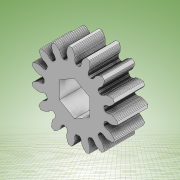
# Autodesk Inventor part: Piñon1
Saved by Autodesk Inventor 2022 (Build 260153000, 153)
## iProperties
Created: 2022-03-08
Part Number: Piñon1
Material: Genérico
Document SubType Name: Modeling
Designer: Marco
Density: 1 g/cm^3
Appearance: Valor por defecto
Author: Marco
Autodesk Inventor part; units mm, degrees
ref_plane "YZ Plane" through (0, 0, 0) normal (1, 0, 0) x (0, 1, 0)
ref_plane "XZ Plane" through (0, 0, 0) normal (0, 1, 0) x (-1, 0, 0)
ref_plane "XY Plane" through (0, 0, 0) normal (0, 0, 1) x (1, 0, 0)
sketch "Boceto1" plane through (0, 0, 0) normal (0, 0, 1) x (1, 0, 0)
  line L0 (7.7848, 3.0032) -> (7.6735, 2.8594)
  line L1 (7.6735, 2.8594) -> (7.565, 2.7306)
  line L2 (7.565, 2.7306) -> (7.4594, 2.6156)
  line L3 (7.4594, 2.6156) -> (7.3576, 2.5136)
  line L4 (7.3576, 2.5136) -> (7.2614, 2.4249)
  line L5 (7.2614, 2.4249) -> (7.1696, 2.3471)
  line L6 (7.1696, 2.3471) -> (7.0863, 2.2824)
  line L7 (7.0863, 2.2824) -> (7.01, 2.228)
  line L8 (7.01, 2.228) -> (6.8817, 2.1478)
  line L9 (6.8817, 2.1478) -> (6.7742, 2.0935)
  line L10 (6.7742, 2.0935) -> (6.6296, 2.0713)
  line L11 (6.6296, 2.0713) -> (6.4798, 2.0382)
  line L12 (6.4798, 2.0382) -> (6.3445, 1.9967)
  line L13 (6.3445, 1.9967) -> (6.2241, 1.948)
  line L14 (6.2241, 1.948) -> (6.119, 1.8933)
  line L15 (6.119, 1.8933) -> (6.0294, 1.8338)
  line L16 (6.0294, 1.8338) -> (5.9556, 1.7706)
  line L17 (5.9556, 1.7706) -> (5.9246, 1.738)
  line L18 (5.9246, 1.738) -> (5.8976, 1.705)
  line L19 (5.8976, 1.705) -> (5.8746, 1.6717)
  line L20 (5.8746, 1.6717) -> (5.8555, 1.6382)
  line L21 (5.8555, 1.6382) -> (5.8404, 1.6048)
  line L22 (5.8404, 1.6048) -> (5.8293, 1.5715)
  line L23 (5.8293, 1.5715) -> (5.8221, 1.5384)
  line L24 (5.8221, 1.5384) -> (5.8189, 1.5059)
  line L25 (5.8189, 1.5059) -> (5.8195, 1.474)
  line L26 (5.8195, 1.474) -> (5.8258, 1.4351)
  line L27 (5.8258, 1.4351) -> (5.8688, 1.2477)
  line L28 (5.8688, 1.2477) -> (5.9058, 1.0589)
  line L29 (5.9058, 1.0589) -> (5.9159, 1.0209)
  line L30 (5.9159, 1.0209) -> (5.9283, 0.9915)
  line L31 (5.9283, 0.9915) -> (5.9445, 0.9631)
  line L32 (5.9445, 0.9631) -> (5.9644, 0.9358)
  line L33 (5.9644, 0.9358) -> (5.9882, 0.9099)
  line L34 (5.9882, 0.9099) -> (6.0156, 0.8855)
  line L35 (6.0156, 0.8855) -> (6.0466, 0.8627)
  line L36 (6.0466, 0.8627) -> (6.0812, 0.8416)
  line L37 (6.0812, 0.8416) -> (6.1193, 0.8224)
  line L38 (6.1193, 0.8224) -> (6.1608, 0.8053)
  line L39 (6.1608, 0.8053) -> (6.254, 0.7776)
  line L40 (6.254, 0.7776) -> (6.36, 0.7597)
  line L41 (6.36, 0.7597) -> (6.4783, 0.7524)
  line L42 (6.4783, 0.7524) -> (6.6081, 0.7569)
  line L43 (6.6081, 0.7569) -> (6.7485, 0.7741)
  line L44 (6.7485, 0.7741) -> (6.8988, 0.8048)
  line L45 (6.8988, 0.8048) -> (7.04, 0.8433)
  line L46 (7.04, 0.8433) -> (7.1603, 0.8374)
  line L47 (7.1603, 0.8374) -> (7.3101, 0.8164)
  line L48 (7.3101, 0.8164) -> (7.4019, 0.7977)
  line L49 (7.4019, 0.7977) -> (7.5044, 0.7724)
  line L50 (7.5044, 0.7724) -> (7.6198, 0.7388)
  line L51 (7.6198, 0.7388) -> (7.7438, 0.6969)
  line L52 (7.7438, 0.6969) -> (7.8783, 0.6451)
  line L53 (7.8783, 0.6451) -> (8.0216, 0.5829)
  line L54 (8.0216, 0.5829) -> (8.1731, 0.5095)
  line L55 (8.1731, 0.5095) -> (8.3334, 0.4231)
  line L56 (8.3334, 0.4231) -> (8.4936, 0.328)
  arc A0 (8.4936, -0.328) -> (8.4936, 0.328) centre (0, 0) ccw
  line L57 (8.4936, -0.328) -> (8.3332, -0.4231)
  line L58 (8.3332, -0.4231) -> (8.1741, -0.5093)
  line L59 (8.1741, -0.5093) -> (8.0225, -0.5827)
  line L60 (8.0225, -0.5827) -> (7.8793, -0.6449)
  line L61 (7.8793, -0.6449) -> (7.7448, -0.6966)
  line L62 (7.7448, -0.6966) -> (7.6208, -0.7384)
  line L63 (7.6208, -0.7384) -> (7.5053, -0.7721)
  line L64 (7.5053, -0.7721) -> (7.4028, -0.7973)
  line L65 (7.4028, -0.7973) -> (7.311, -0.8159)
  line L66 (7.311, -0.8159) -> (7.1612, -0.8369)
  line L67 (7.1612, -0.8369) -> (7.0409, -0.8427)
  line L68 (7.0409, -0.8427) -> (6.8997, -0.8042)
  line L69 (6.8997, -0.8042) -> (6.7494, -0.7734)
  line L70 (6.7494, -0.7734) -> (6.609, -0.7562)
  line L71 (6.609, -0.7562) -> (6.4792, -0.7517)
  line L72 (6.4792, -0.7517) -> (6.361, -0.7589)
  line L73 (6.361, -0.7589) -> (6.2549, -0.7768)
  line L74 (6.2549, -0.7768) -> (6.1617, -0.8044)
  line L75 (6.1617, -0.8044) -> (6.1202, -0.8216)
  line L76 (6.1202, -0.8216) -> (6.0821, -0.8407)
  line L77 (6.0821, -0.8407) -> (6.0475, -0.8618)
  line L78 (6.0475, -0.8618) -> (6.0164, -0.8846)
  line L79 (6.0164, -0.8846) -> (5.989, -0.909)
  line L80 (5.989, -0.909) -> (5.9653, -0.9349)
  line L81 (5.9653, -0.9349) -> (5.9453, -0.9621)
  line L82 (5.9453, -0.9621) -> (5.9291, -0.9906)
  line L83 (5.9291, -0.9906) -> (5.9167, -1.02)
  line L84 (5.9167, -1.02) -> (5.9066, -1.058)
  line L85 (5.9066, -1.058) -> (5.8696, -1.2467)
  line L86 (5.8696, -1.2467) -> (5.8265, -1.4342)
  line L87 (5.8265, -1.4342) -> (5.8202, -1.473)
  line L88 (5.8202, -1.473) -> (5.8196, -1.5049)
  line L89 (5.8196, -1.5049) -> (5.8228, -1.5375)
  line L90 (5.8228, -1.5375) -> (5.83, -1.5705)
  line L91 (5.83, -1.5705) -> (5.8411, -1.6038)
  line L92 (5.8411, -1.6038) -> (5.8561, -1.6373)
  line L93 (5.8561, -1.6373) -> (5.8752, -1.6708)
  line L94 (5.8752, -1.6708) -> (5.8982, -1.7041)
  line L95 (5.8982, -1.7041) -> (5.9252, -1.7371)
  line L96 (5.9252, -1.7371) -> (5.9562, -1.7697)
  line L97 (5.9562, -1.7697) -> (6.03, -1.8329)
  line L98 (6.03, -1.8329) -> (6.1196, -1.8925)
  line L99 (6.1196, -1.8925) -> (6.2246, -1.9472)
  line L100 (6.2246, -1.9472) -> (6.345, -1.9959)
  line L101 (6.345, -1.9959) -> (6.4803, -2.0374)
  line L102 (6.4803, -2.0374) -> (6.63, -2.0706)
  line L103 (6.63, -2.0706) -> (6.7746, -2.0929)
  line L104 (6.7746, -2.0929) -> (6.8822, -2.1472)
  line L105 (6.8822, -2.1472) -> (7.0104, -2.2275)
  line L106 (7.0104, -2.2275) -> (7.0867, -2.2818)
  line L107 (7.0867, -2.2818) -> (7.17, -2.3467)
  line L108 (7.17, -2.3467) -> (7.2617, -2.4244)
  line L109 (7.2617, -2.4244) -> (7.3579, -2.5131)
  line L110 (7.3579, -2.5131) -> (7.4597, -2.6152)
  line L111 (7.4597, -2.6152) -> (7.5652, -2.7303)
  line L112 (7.5652, -2.7303) -> (7.6737, -2.859)
  line L113 (7.6737, -2.859) -> (7.785, -3.0029)
  line L114 (7.785, -3.0029) -> (7.8927, -3.155)
  arc A1 (7.6259, -3.7544) -> (7.8927, -3.155) centre (0, 0) ccw
  line L115 (7.6259, -3.7544) -> (7.4407, -3.776)
  line L116 (7.4407, -3.776) -> (7.2594, -3.7895)
  line L117 (7.2594, -3.7895) -> (7.0911, -3.795)
  line L118 (7.0911, -3.795) -> (6.935, -3.7935)
  line L119 (6.935, -3.7935) -> (6.791, -3.7861)
  line L120 (6.791, -3.7861) -> (6.6607, -3.774)
  line L121 (6.6607, -3.774) -> (6.5416, -3.7578)
  line L122 (6.5416, -3.7578) -> (6.4376, -3.7392)
  line L123 (6.4376, -3.7392) -> (6.3462, -3.7189)
  line L124 (6.3462, -3.7189) -> (6.2008, -3.6772)
  line L125 (6.2008, -3.6772) -> (6.0885, -3.6336)
  line L126 (6.0885, -3.6336) -> (5.9752, -3.541)
  line L127 (5.9752, -3.541) -> (5.8504, -3.4518)
  line L128 (5.8504, -3.4518) -> (5.729, -3.379)
  line L129 (5.729, -3.379) -> (5.6123, -3.3222)
  line L130 (5.6123, -3.3222) -> (5.5013, -3.2807)
  line L131 (5.5013, -3.2807) -> (5.3972, -3.2539)
  line L132 (5.3972, -3.2539) -> (5.3008, -3.2413)
  line L133 (5.3008, -3.2413) -> (5.2559, -3.2401)
  line L134 (5.2559, -3.2401) -> (5.2133, -3.2421)
  line L135 (5.2133, -3.2421) -> (5.1731, -3.2473)
  line L136 (5.1731, -3.2473) -> (5.1355, -3.2555)
  line L137 (5.1355, -3.2555) -> (5.1005, -3.2667)
  line L138 (5.1005, -3.2667) -> (5.0683, -3.2807)
  line L139 (5.0683, -3.2807) -> (5.039, -3.2975)
  line L140 (5.039, -3.2975) -> (5.0126, -3.3168)
  line L141 (5.0126, -3.3168) -> (4.9893, -3.3387)
  line L142 (4.9893, -3.3387) -> (4.9646, -3.3693)
  line L143 (4.9646, -3.3693) -> (4.8541, -3.5267)
  line L144 (4.8541, -3.5267) -> (4.7386, -3.6805)
  line L145 (4.7386, -3.6805) -> (4.7171, -3.7134)
  line L146 (4.7171, -3.7134) -> (4.7035, -3.7423)
  line L147 (4.7035, -3.7423) -> (4.6932, -3.7734)
  line L148 (4.6932, -3.7734) -> (4.6863, -3.8064)
  line L149 (4.6863, -3.8064) -> (4.683, -3.8414)
  line L150 (4.683, -3.8414) -> (4.6831, -3.8781)
  line L151 (4.6831, -3.8781) -> (4.6869, -3.9164)
  line L152 (4.6869, -3.9164) -> (4.6944, -3.9562)
  line L153 (4.6944, -3.9562) -> (4.7057, -3.9974)
  line L154 (4.7057, -3.9974) -> (4.7207, -4.0397)
  line L155 (4.7207, -4.0397) -> (4.7625, -4.1275)
  line L156 (4.7625, -4.1275) -> (4.8201, -4.2183)
  line L157 (4.8201, -4.2183) -> (4.8939, -4.311)
  line L158 (4.8939, -4.311) -> (4.984, -4.4045)
  line L159 (4.984, -4.4045) -> (5.0908, -4.4974)
  line L160 (5.0908, -4.4974) -> (5.2141, -4.5885)
  line L161 (5.2141, -4.5885) -> (5.3372, -4.6677)
  line L162 (5.3372, -4.6677) -> (5.4134, -4.761)
  line L163 (5.4134, -4.761) -> (5.498, -4.8864)
  line L164 (5.498, -4.8864) -> (5.5455, -4.9671)
  line L165 (5.5455, -4.9671) -> (5.5953, -5.0602)
  line L166 (5.5953, -5.0602) -> (5.6475, -5.1685)
  line L167 (5.6475, -5.1685) -> (5.6994, -5.2887)
  line L168 (5.6994, -5.2887) -> (5.7509, -5.4233)
  line L169 (5.7509, -5.4233) -> (5.8005, -5.5713)
  line L170 (5.8005, -5.5713) -> (5.8473, -5.7331)
  line L171 (5.8473, -5.7331) -> (5.8905, -5.9097)
  line L172 (5.8905, -5.9097) -> (5.9271, -6.0925)
  arc A2 (5.4396, -6.5315) -> (5.9271, -6.0925) centre (0, 0) ccw
  line L173 (5.4396, -6.5315) -> (5.2616, -6.4759)
  line L174 (5.2616, -6.4759) -> (5.0905, -6.4145)
  line L175 (5.0905, -6.4145) -> (4.9345, -6.3511)
  line L176 (4.9345, -6.3511) -> (4.7924, -6.2862)
  line L177 (4.7924, -6.2862) -> (4.664, -6.221)
  line L178 (4.664, -6.221) -> (4.5499, -6.1568)
  line L179 (4.5499, -6.1568) -> (4.4476, -6.0936)
  line L180 (4.4476, -6.0936) -> (4.3602, -6.0343)
  line L181 (4.3602, -6.0343) -> (4.285, -5.9786)
  line L182 (4.285, -5.9786) -> (4.1691, -5.8814)
  line L183 (4.1691, -5.8814) -> (4.0842, -5.7958)
  line L184 (4.0842, -5.7958) -> (4.0184, -5.6652)
  line L185 (4.0184, -5.6652) -> (3.9406, -5.533)
  line L186 (3.9406, -5.533) -> (3.8594, -5.4171)
  line L187 (3.8594, -5.4171) -> (3.7759, -5.3177)
  line L188 (3.7759, -5.3177) -> (3.6914, -5.2346)
  line L189 (3.6914, -5.2346) -> (3.6071, -5.1678)
  line L190 (3.6071, -5.1678) -> (3.5242, -5.1171)
  line L191 (3.5242, -5.1171) -> (3.4836, -5.0977)
  line L192 (3.4836, -5.0977) -> (3.4439, -5.0822)
  line L193 (3.4439, -5.0822) -> (3.4051, -5.0706)
  line L194 (3.4051, -5.0706) -> (3.3673, -5.0628)
  line L195 (3.3673, -5.0628) -> (3.3309, -5.0588)
  line L196 (3.3309, -5.0588) -> (3.2957, -5.0585)
  line L197 (3.2957, -5.0585) -> (3.2621, -5.0619)
  line L198 (3.2621, -5.0619) -> (3.2302, -5.0689)
  line L199 (3.2302, -5.0689) -> (3.2, -5.0794)
  line L200 (3.2, -5.0794) -> (3.165, -5.0973)
  line L201 (3.165, -5.0973) -> (3, -5.1961)
  line L202 (3, -5.1961) -> (2.8319, -5.2896)
  line L203 (2.8319, -5.2896) -> (2.7989, -5.311)
  line L204 (2.7989, -5.311) -> (2.7747, -5.3318)
  line L205 (2.7747, -5.3318) -> (2.7527, -5.356)
  line L206 (2.7527, -5.356) -> (2.733, -5.3835)
  line L207 (2.733, -5.3835) -> (2.7157, -5.414)
  line L208 (2.7157, -5.414) -> (2.7009, -5.4476)
  line L209 (2.7009, -5.4476) -> (2.6888, -5.4842)
  line L210 (2.6888, -5.4842) -> (2.6794, -5.5236)
  line L211 (2.6794, -5.5236) -> (2.673, -5.5658)
  line L212 (2.673, -5.5658) -> (2.6695, -5.6106)
  line L213 (2.6695, -5.6106) -> (2.6719, -5.7077)
  line L214 (2.6719, -5.7077) -> (2.6876, -5.8141)
  line L215 (2.6876, -5.8141) -> (2.7173, -5.9288)
  line L216 (2.7173, -5.9288) -> (2.7617, -6.0509)
  line L217 (2.7617, -6.0509) -> (2.8214, -6.1791)
  line L218 (2.8214, -6.1791) -> (2.8971, -6.3126)
  line L219 (2.8971, -6.3126) -> (2.9773, -6.4349)
  line L220 (2.9773, -6.4349) -> (3.0089, -6.5512)
  line L221 (3.0089, -6.5512) -> (3.0352, -6.7002)
  line L222 (3.0352, -6.7002) -> (3.0458, -6.7932)
  line L223 (3.0458, -6.7932) -> (3.0534, -6.8985)
  line L224 (3.0534, -6.8985) -> (3.0571, -7.0187)
  line L225 (3.0571, -7.0187) -> (3.0555, -7.1496)
  line L226 (3.0555, -7.1496) -> (3.0478, -7.2935)
  line L227 (3.0478, -7.2935) -> (3.033, -7.449)
  line L228 (3.033, -7.449) -> (3.0099, -7.6157)
  line L229 (3.0099, -7.6157) -> (2.9775, -7.7947)
  line L230 (2.9775, -7.7947) -> (2.9366, -7.9766)
  arc A3 (2.3127, -8.1793) -> (2.9366, -7.9766) centre (0, 0) ccw
  line L231 (2.3127, -8.1793) -> (2.1727, -8.0562)
  line L232 (2.1727, -8.0562) -> (2.0413, -7.9305)
  line L233 (2.0413, -7.9305) -> (1.9247, -7.8092)
  line L234 (1.9247, -7.8092) -> (1.8213, -7.6921)
  line L235 (1.8213, -7.6921) -> (1.7305, -7.5802)
  line L236 (1.7305, -7.5802) -> (1.6523, -7.4752)
  line L237 (1.6523, -7.4752) -> (1.5846, -7.3758)
  line L238 (1.5846, -7.3758) -> (1.5289, -7.2862)
  line L239 (1.5289, -7.2862) -> (1.4828, -7.2047)
  line L240 (1.4828, -7.2047) -> (1.4165, -7.0687)
  line L241 (1.4165, -7.0687) -> (1.3737, -6.956)
  line L242 (1.3737, -6.956) -> (1.3667, -6.8099)
  line L243 (1.3667, -6.8099) -> (1.3495, -6.6575)
  line L244 (1.3495, -6.6575) -> (1.3224, -6.5186)
  line L245 (1.3224, -6.5186) -> (1.2866, -6.3938)
  line L246 (1.2866, -6.3938) -> (1.2432, -6.2835)
  line L247 (1.2432, -6.2835) -> (1.1933, -6.1882)
  line L248 (1.1933, -6.1882) -> (1.1382, -6.1082)
  line L249 (1.1382, -6.1082) -> (1.1091, -6.074)
  line L250 (1.1091, -6.074) -> (1.0791, -6.0437)
  line L251 (1.0791, -6.0437) -> (1.0483, -6.0173)
  line L252 (1.0483, -6.0173) -> (1.017, -5.9948)
  line L253 (1.017, -5.9948) -> (0.9853, -5.9763)
  line L254 (0.9853, -5.9763) -> (0.9534, -5.9618)
  line L255 (0.9534, -5.9618) -> (0.9213, -5.9512)
  line L256 (0.9213, -5.9512) -> (0.8893, -5.9445)
  line L257 (0.8893, -5.9445) -> (0.8575, -5.9418)
  line L258 (0.8575, -5.9418) -> (0.8182, -5.944)
  line L259 (0.8182, -5.944) -> (0.6272, -5.9672)
  line L260 (0.6272, -5.9672) -> (0.4357, -5.9842)
  line L261 (0.4357, -5.9842) -> (0.3968, -5.9902)
  line L262 (0.3968, -5.9902) -> (0.3662, -5.9995)
  line L263 (0.3662, -5.9995) -> (0.3363, -6.0126)
  line L264 (0.3363, -6.0126) -> (0.3071, -6.0297)
  line L265 (0.3071, -6.0297) -> (0.2789, -6.0505)
  line L266 (0.2789, -6.0505) -> (0.2517, -6.0752)
  line L267 (0.2517, -6.0752) -> (0.2258, -6.1037)
  line L268 (0.2258, -6.1037) -> (0.2012, -6.1359)
  line L269 (0.2012, -6.1359) -> (0.1781, -6.1718)
  line L270 (0.1781, -6.1718) -> (0.1567, -6.2113)
  line L271 (0.1567, -6.2113) -> (0.1195, -6.301)
  line L272 (0.1195, -6.301) -> (0.0905, -6.4046)
  line L273 (0.0905, -6.4046) -> (0.071, -6.5215)
  line L274 (0.071, -6.5215) -> (0.0619, -6.651)
  line L275 (0.0619, -6.651) -> (0.0642, -6.7925)
  line L276 (0.0642, -6.7925) -> (0.079, -6.9452)
  line L277 (0.079, -6.9452) -> (0.1026, -7.0896)
  line L278 (0.1026, -7.0896) -> (0.0842, -7.2086)
  line L279 (0.0842, -7.2086) -> (0.0475, -7.3555)
  line L280 (0.0475, -7.3555) -> (0.0194, -7.4448)
  line L281 (0.0194, -7.4448) -> (-0.0165, -7.544)
  line L282 (-0.0165, -7.544) -> (-0.062, -7.6554)
  line L283 (-0.062, -7.6554) -> (-0.1166, -7.7743)
  line L284 (-0.1166, -7.7743) -> (-0.1822, -7.9026)
  line L285 (-0.1822, -7.9026) -> (-0.259, -8.0386)
  line L286 (-0.259, -8.0386) -> (-0.3479, -8.1816)
  line L287 (-0.3479, -8.1816) -> (-0.4503, -8.3319)
  line L288 (-0.4503, -8.3319) -> (-0.5616, -8.4814)
  arc A4 (-1.214, -8.4128) -> (-0.5616, -8.4814) centre (0, 0) ccw
  line L289 (-1.214, -8.4128) -> (-1.2918, -8.2434)
  line L290 (-1.2918, -8.2434) -> (-1.3607, -8.0751)
  line L291 (-1.3607, -8.0751) -> (-1.4179, -7.9168)
  line L292 (-1.4179, -7.9168) -> (-1.4648, -7.7678)
  line L293 (-1.4648, -7.7678) -> (-1.5023, -7.6286)
  line L294 (-1.5023, -7.6286) -> (-1.531, -7.501)
  line L295 (-1.531, -7.501) -> (-1.5524, -7.3826)
  line L296 (-1.5524, -7.3826) -> (-1.5668, -7.278)
  line L297 (-1.5668, -7.278) -> (-1.5758, -7.1848)
  line L298 (-1.5758, -7.1848) -> (-1.581, -7.0336)
  line L299 (-1.581, -7.0336) -> (-1.5743, -6.9133)
  line L300 (-1.5743, -6.9133) -> (-1.5213, -6.777)
  line L301 (-1.5213, -6.777) -> (-1.475, -6.6307)
  line L302 (-1.475, -6.6307) -> (-1.4433, -6.4928)
  line L303 (-1.4433, -6.4928) -> (-1.4253, -6.3642)
  line L304 (-1.4253, -6.3642) -> (-1.4201, -6.2459)
  line L305 (-1.4201, -6.2459) -> (-1.4268, -6.1385)
  line L306 (-1.4268, -6.1385) -> (-1.4446, -6.043)
  line L307 (-1.4446, -6.043) -> (-1.4573, -5.9999)
  line L308 (-1.4573, -5.9999) -> (-1.4724, -5.96)
  line L309 (-1.4724, -5.96) -> (-1.4898, -5.9234)
  line L310 (-1.4898, -5.9234) -> (-1.5092, -5.8901)
  line L311 (-1.5092, -5.8901) -> (-1.5307, -5.8603)
  line L312 (-1.5307, -5.8603) -> (-1.554, -5.834)
  line L313 (-1.554, -5.834) -> (-1.5789, -5.8113)
  line L314 (-1.5789, -5.8113) -> (-1.6055, -5.7922)
  line L315 (-1.6055, -5.7922) -> (-1.6335, -5.7768)
  line L316 (-1.6335, -5.7768) -> (-1.6703, -5.7628)
  line L317 (-1.6703, -5.7628) -> (-1.8541, -5.7063)
  line L318 (-1.8541, -5.7063) -> (-2.036, -5.644)
  line L319 (-2.036, -5.644) -> (-2.074, -5.6337)
  line L320 (-2.074, -5.6337) -> (-2.1057, -5.6297)
  line L321 (-2.1057, -5.6297) -> (-2.1384, -5.6295)
  line L322 (-2.1384, -5.6295) -> (-2.172, -5.6332)
  line L323 (-2.172, -5.6332) -> (-2.2063, -5.6408)
  line L324 (-2.2063, -5.6408) -> (-2.2411, -5.6523)
  line L325 (-2.2411, -5.6523) -> (-2.2764, -5.6678)
  line L326 (-2.2764, -5.6678) -> (-2.3119, -5.6872)
  line L327 (-2.3119, -5.6872) -> (-2.3476, -5.7106)
  line L328 (-2.3476, -5.7106) -> (-2.3832, -5.738)
  line L329 (-2.3832, -5.738) -> (-2.4538, -5.8049)
  line L330 (-2.4538, -5.8049) -> (-2.5223, -5.8877)
  line L331 (-2.5223, -5.8877) -> (-2.5877, -5.9865)
  line L332 (-2.5877, -5.9865) -> (-2.6487, -6.1012)
  line L333 (-2.6487, -6.1012) -> (-2.7041, -6.2314)
  line L334 (-2.7041, -6.2314) -> (-2.7527, -6.3769)
  line L335 (-2.7527, -6.3769) -> (-2.7899, -6.5184)
  line L336 (-2.7899, -6.5184) -> (-2.8552, -6.6196)
  line L337 (-2.8552, -6.6196) -> (-2.9483, -6.7389)
  line L338 (-2.9483, -6.7389) -> (-3.0103, -6.809)
  line L339 (-3.0103, -6.809) -> (-3.0835, -6.8851)
  line L340 (-3.0835, -6.8851) -> (-3.1704, -6.9683)
  line L341 (-3.1704, -6.9683) -> (-3.2686, -7.0547)
  line L342 (-3.2686, -7.0547) -> (-3.3807, -7.1453)
  line L343 (-3.3807, -7.1453) -> (-3.5062, -7.2383)
  line L344 (-3.5062, -7.2383) -> (-3.6456, -7.3327)
  line L345 (-3.6456, -7.3327) -> (-3.8002, -7.4284)
  line L346 (-3.8002, -7.4284) -> (-3.9628, -7.5197)
  arc A5 (-4.5309, -7.1917) -> (-3.9628, -7.5197) centre (0, 0) ccw
  line L347 (-4.5309, -7.1917) -> (-4.533, -7.0053)
  line L348 (-4.533, -7.0053) -> (-4.5275, -6.8235)
  line L349 (-4.5275, -6.8235) -> (-4.5154, -6.6556)
  line L350 (-4.5154, -6.6556) -> (-4.4976, -6.5004)
  line L351 (-4.4976, -6.5004) -> (-4.4752, -6.3581)
  line L352 (-4.4752, -6.3581) -> (-4.4495, -6.2298)
  line L353 (-4.4495, -6.2298) -> (-4.4209, -6.1129)
  line L354 (-4.4209, -6.1129) -> (-4.3916, -6.0115)
  line L355 (-4.3916, -6.0115) -> (-4.3619, -5.9228)
  line L356 (-4.3619, -5.9228) -> (-4.3052, -5.7825)
  line L357 (-4.3052, -5.7825) -> (-4.2501, -5.6753)
  line L358 (-4.2501, -5.6753) -> (-4.1462, -5.5723)
  line L359 (-4.1462, -5.5723) -> (-4.0444, -5.4575)
  line L360 (-4.0444, -5.4575) -> (-3.9594, -5.3445)
  line L361 (-3.9594, -5.3445) -> (-3.8906, -5.2343)
  line L362 (-3.8906, -5.2343) -> (-3.8377, -5.1283)
  line L363 (-3.8377, -5.1283) -> (-3.8002, -5.0275)
  line L364 (-3.8002, -5.0275) -> (-3.7776, -4.933)
  line L365 (-3.7776, -4.933) -> (-3.7717, -4.8884)
  line L366 (-3.7717, -4.8884) -> (-3.7693, -4.8458)
  line L367 (-3.7693, -4.8458) -> (-3.7702, -4.8053)
  line L368 (-3.7702, -4.8053) -> (-3.7745, -4.7671)
  line L369 (-3.7745, -4.7671) -> (-3.7819, -4.7311)
  line L370 (-3.7819, -4.7311) -> (-3.7925, -4.6976)
  line L371 (-3.7925, -4.6976) -> (-3.8061, -4.6667)
  line L372 (-3.8061, -4.6667) -> (-3.8226, -4.6385)
  line L373 (-3.8226, -4.6385) -> (-3.8419, -4.613)
  line L374 (-3.8419, -4.613) -> (-3.8698, -4.5853)
  line L375 (-3.8698, -4.5853) -> (-4.0148, -4.4589)
  line L376 (-4.0148, -4.4589) -> (-4.1556, -4.3279)
  line L377 (-4.1556, -4.3279) -> (-4.1861, -4.3031)
  line L378 (-4.1861, -4.3031) -> (-4.2134, -4.2865)
  line L379 (-4.2134, -4.2865) -> (-4.2433, -4.2731)
  line L380 (-4.2433, -4.2731) -> (-4.2754, -4.2628)
  line L381 (-4.2754, -4.2628) -> (-4.3098, -4.2558)
  line L382 (-4.3098, -4.2558) -> (-4.3464, -4.2521)
  line L383 (-4.3464, -4.2521) -> (-4.3849, -4.2519)
  line L384 (-4.3849, -4.2519) -> (-4.4253, -4.2552)
  line L385 (-4.4253, -4.2552) -> (-4.4674, -4.2621)
  line L386 (-4.4674, -4.2621) -> (-4.511, -4.2726)
  line L387 (-4.511, -4.2726) -> (-4.6027, -4.305)
  line L388 (-4.6027, -4.305) -> (-4.699, -4.3528)
  line L389 (-4.699, -4.3528) -> (-4.799, -4.4165)
  line L390 (-4.799, -4.4165) -> (-4.9013, -4.4964)
  line L391 (-4.9013, -4.4964) -> (-5.0048, -4.5928)
  line L392 (-5.0048, -4.5928) -> (-5.1084, -4.706)
  line L393 (-5.1084, -4.706) -> (-5.2, -4.8201)
  line L394 (-5.2, -4.8201) -> (-5.3008, -4.8861)
  line L395 (-5.3008, -4.8861) -> (-5.4343, -4.9571)
  line L396 (-5.4343, -4.9571) -> (-5.5195, -4.9959)
  line L397 (-5.5195, -4.9959) -> (-5.6173, -5.0357)
  line L398 (-5.6173, -5.0357) -> (-5.7305, -5.0764)
  line L399 (-5.7305, -5.0764) -> (-5.8554, -5.1153)
  line L400 (-5.8554, -5.1153) -> (-5.9947, -5.1525)
  line L401 (-5.9947, -5.1525) -> (-6.1471, -5.1864)
  line L402 (-6.1471, -5.1864) -> (-6.3129, -5.216)
  line L403 (-6.3129, -5.216) -> (-6.4931, -5.2405)
  line L404 (-6.4931, -5.2405) -> (-6.6787, -5.2578)
  arc A6 (-7.0643, -4.7271) -> (-6.6787, -5.2578) centre (0, 0) ccw
  line L405 (-7.0643, -4.7271) -> (-6.9905, -4.5559)
  line L406 (-6.9905, -4.5559) -> (-6.9115, -4.3921)
  line L407 (-6.9115, -4.3921) -> (-6.8321, -4.2436)
  line L408 (-6.8321, -4.2436) -> (-6.7528, -4.1091)
  line L409 (-6.7528, -4.1091) -> (-6.6744, -3.9881)
  line L410 (-6.6744, -3.9881) -> (-6.5987, -3.8814)
  line L411 (-6.5987, -3.8814) -> (-6.5251, -3.7863)
  line L412 (-6.5251, -3.7863) -> (-6.457, -3.7056)
  line L413 (-6.457, -3.7056) -> (-6.3938, -3.6366)
  line L414 (-6.3938, -3.6366) -> (-6.2849, -3.5315)
  line L415 (-6.2849, -3.5315) -> (-6.191, -3.456)
  line L416 (-6.191, -3.456) -> (-6.0542, -3.4042)
  line L417 (-6.0542, -3.4042) -> (-5.9146, -3.3407)
  line L418 (-5.9146, -3.3407) -> (-5.7909, -3.272)
  line L419 (-5.7909, -3.272) -> (-5.6832, -3.1993)
  line L420 (-5.6832, -3.1993) -> (-5.5918, -3.124)
  line L421 (-5.5918, -3.124) -> (-5.5166, -3.0471)
  line L422 (-5.5166, -3.0471) -> (-5.4575, -2.97)
  line L423 (-5.4575, -2.97) -> (-5.4339, -2.9317)
  line L424 (-5.4339, -2.9317) -> (-5.4144, -2.8938)
  line L425 (-5.4144, -2.8938) -> (-5.3988, -2.8564)
  line L426 (-5.3988, -2.8564) -> (-5.3871, -2.8197)
  line L427 (-5.3871, -2.8197) -> (-5.3793, -2.7838)
  line L428 (-5.3793, -2.7838) -> (-5.3753, -2.7489)
  line L429 (-5.3753, -2.7489) -> (-5.3752, -2.7151)
  line L430 (-5.3752, -2.7151) -> (-5.3788, -2.6826)
  line L431 (-5.3788, -2.6826) -> (-5.386, -2.6515)
  line L432 (-5.386, -2.6515) -> (-5.4002, -2.6148)
  line L433 (-5.4002, -2.6148) -> (-5.4813, -2.4404)
  line L434 (-5.4813, -2.4404) -> (-5.5567, -2.2635)
  line L435 (-5.5567, -2.2635) -> (-5.5744, -2.2284)
  line L436 (-5.5744, -2.2284) -> (-5.5927, -2.2022)
  line L437 (-5.5927, -2.2022) -> (-5.6144, -2.1778)
  line L438 (-5.6144, -2.1778) -> (-5.6396, -2.1553)
  line L439 (-5.6396, -2.1553) -> (-5.6682, -2.1349)
  line L440 (-5.6682, -2.1349) -> (-5.7001, -2.1167)
  line L441 (-5.7001, -2.1167) -> (-5.7352, -2.1008)
  line L442 (-5.7352, -2.1008) -> (-5.7734, -2.0874)
  line L443 (-5.7734, -2.0874) -> (-5.8147, -2.0765)
  line L444 (-5.8147, -2.0765) -> (-5.8589, -2.0684)
  line L445 (-5.8589, -2.0684) -> (-5.9557, -2.0607)
  line L446 (-5.9557, -2.0607) -> (-6.0632, -2.0652)
  line L447 (-6.0632, -2.0652) -> (-6.1804, -2.0827)
  line L448 (-6.1804, -2.0827) -> (-6.3064, -2.1141)
  line L449 (-6.3064, -2.1141) -> (-6.4402, -2.16)
  line L450 (-6.4402, -2.16) -> (-6.5808, -2.2213)
  line L451 (-6.5808, -2.2213) -> (-6.7109, -2.2883)
  line L452 (-6.7109, -2.2883) -> (-6.8298, -2.3076)
  line L453 (-6.8298, -2.3076) -> (-6.9808, -2.3182)
  line L454 (-6.9808, -2.3182) -> (-7.0744, -2.319)
  line L455 (-7.0744, -2.319) -> (-7.1799, -2.3156)
  line L456 (-7.1799, -2.3156) -> (-7.2998, -2.3066)
  line L457 (-7.2998, -2.3066) -> (-7.4298, -2.2915)
  line L458 (-7.4298, -2.2915) -> (-7.5721, -2.2688)
  line L459 (-7.5721, -2.2688) -> (-7.7252, -2.2377)
  line L460 (-7.7252, -2.2377) -> (-7.8886, -2.1974)
  line L461 (-7.8886, -2.1974) -> (-8.0632, -2.1464)
  line L462 (-8.0632, -2.1464) -> (-8.2398, -2.0868)
  arc A7 (-8.3767, -1.4422) -> (-8.2398, -2.0868) centre (0, 0) ccw
  line L463 (-8.3767, -1.4422) -> (-8.2397, -1.3158)
  line L464 (-8.2397, -1.3158) -> (-8.1009, -1.1983)
  line L465 (-8.1009, -1.1983) -> (-7.968, -1.095)
  line L466 (-7.968, -1.095) -> (-7.8407, -1.0044)
  line L467 (-7.8407, -1.0044) -> (-7.72, -0.9258)
  line L468 (-7.72, -0.9258) -> (-7.6074, -0.8591)
  line L469 (-7.6074, -0.8591) -> (-7.5014, -0.8022)
  line L470 (-7.5014, -0.8022) -> (-7.4064, -0.7562)
  line L471 (-7.4064, -0.7562) -> (-7.3205, -0.7189)
  line L472 (-7.3205, -0.7189) -> (-7.1783, -0.6672)
  line L473 (-7.1783, -0.6672) -> (-7.0618, -0.6365)
  line L474 (-7.0618, -0.6365) -> (-6.9157, -0.6449)
  line L475 (-6.9157, -0.6449) -> (-6.7623, -0.6437)
  line L476 (-6.7623, -0.6437) -> (-6.6214, -0.6314)
  line L477 (-6.6214, -0.6314) -> (-6.4935, -0.6088)
  line L478 (-6.4935, -0.6088) -> (-6.3793, -0.5772)
  line L479 (-6.3793, -0.5772) -> (-6.2793, -0.5377)
  line L480 (-6.2793, -0.5377) -> (-6.1939, -0.4913)
  line L481 (-6.1939, -0.4913) -> (-6.1568, -0.4659)
  line L482 (-6.1568, -0.4659) -> (-6.1235, -0.4392)
  line L483 (-6.1235, -0.4392) -> (-6.0941, -0.4114)
  line L484 (-6.0941, -0.4114) -> (-6.0684, -0.3826)
  line L485 (-6.0684, -0.3826) -> (-6.0467, -0.3531)
  line L486 (-6.0467, -0.3531) -> (-6.0289, -0.3228)
  line L487 (-6.0289, -0.3228) -> (-6.015, -0.292)
  line L488 (-6.015, -0.292) -> (-6.005, -0.2609)
  line L489 (-6.005, -0.2609) -> (-5.999, -0.2295)
  line L490 (-5.999, -0.2295) -> (-5.9971, -0.1902)
  line L491 (-5.9971, -0.1902) -> (-6.0001, 0.0021)
  line L492 (-6.0001, 0.0021) -> (-5.9969, 0.1944)
  line L493 (-5.9969, 0.1944) -> (-5.9988, 0.2337)
  line L494 (-5.9988, 0.2337) -> (-6.0048, 0.2651)
  line L495 (-6.0048, 0.2651) -> (-6.0147, 0.2962)
  line L496 (-6.0147, 0.2962) -> (-6.0286, 0.327)
  line L497 (-6.0286, 0.327) -> (-6.0464, 0.3573)
  line L498 (-6.0464, 0.3573) -> (-6.0681, 0.3869)
  line L499 (-6.0681, 0.3869) -> (-6.0937, 0.4157)
  line L500 (-6.0937, 0.4157) -> (-6.1231, 0.4435)
  line L501 (-6.1231, 0.4435) -> (-6.1564, 0.4702)
  line L502 (-6.1564, 0.4702) -> (-6.1935, 0.4956)
  line L503 (-6.1935, 0.4956) -> (-6.2788, 0.5421)
  line L504 (-6.2788, 0.5421) -> (-6.3788, 0.5818)
  line L505 (-6.3788, 0.5818) -> (-6.493, 0.6135)
  line L506 (-6.493, 0.6135) -> (-6.6208, 0.6361)
  line L507 (-6.6208, 0.6361) -> (-6.7618, 0.6486)
  line L508 (-6.7618, 0.6486) -> (-6.9152, 0.6499)
  line L509 (-6.9152, 0.6499) -> (-7.0612, 0.6417)
  line L510 (-7.0612, 0.6417) -> (-7.1777, 0.6725)
  line L511 (-7.1777, 0.6725) -> (-7.3199, 0.7243)
  line L512 (-7.3199, 0.7243) -> (-7.4057, 0.7616)
  line L513 (-7.4057, 0.7616) -> (-7.5007, 0.8077)
  line L514 (-7.5007, 0.8077) -> (-7.6066, 0.8647)
  line L515 (-7.6066, 0.8647) -> (-7.7191, 0.9315)
  line L516 (-7.7191, 0.9315) -> (-7.8399, 1.0102)
  line L517 (-7.8399, 1.0102) -> (-7.9671, 1.1008)
  line L518 (-7.9671, 1.1008) -> (-8.0999, 1.2042)
  line L519 (-8.0999, 1.2042) -> (-8.2387, 1.3218)
  line L520 (-8.2387, 1.3218) -> (-8.3757, 1.4482)
  arc A8 (-8.2391, 2.0897) -> (-8.3757, 1.4482) centre (0, 0) ccw
  line L521 (-8.2391, 2.0897) -> (-8.0625, 2.1493)
  line L522 (-8.0625, 2.1493) -> (-7.8879, 2.2002)
  line L523 (-7.8879, 2.2002) -> (-7.7244, 2.2404)
  line L524 (-7.7244, 2.2404) -> (-7.5713, 2.2714)
  line L525 (-7.5713, 2.2714) -> (-7.429, 2.2941)
  line L526 (-7.429, 2.2941) -> (-7.299, 2.3092)
  line L527 (-7.299, 2.3092) -> (-7.1791, 2.3181)
  line L528 (-7.1791, 2.3181) -> (-7.0736, 2.3215)
  line L529 (-7.0736, 2.3215) -> (-6.9799, 2.3206)
  line L530 (-6.9799, 2.3206) -> (-6.829, 2.31)
  line L531 (-6.829, 2.31) -> (-6.7101, 2.2907)
  line L532 (-6.7101, 2.2907) -> (-6.5801, 2.2237)
  line L533 (-6.5801, 2.2237) -> (-6.4395, 2.1623)
  line L534 (-6.4395, 2.1623) -> (-6.3056, 2.1163)
  line L535 (-6.3056, 2.1163) -> (-6.1797, 2.0849)
  line L536 (-6.1797, 2.0849) -> (-6.0625, 2.0673)
  line L537 (-6.0625, 2.0673) -> (-5.955, 2.0628)
  line L538 (-5.955, 2.0628) -> (-5.8581, 2.0705)
  line L539 (-5.8581, 2.0705) -> (-5.8139, 2.0786)
  line L540 (-5.8139, 2.0786) -> (-5.7727, 2.0894)
  line L541 (-5.7727, 2.0894) -> (-5.7344, 2.1028)
  line L542 (-5.7344, 2.1028) -> (-5.6993, 2.1187)
  line L543 (-5.6993, 2.1187) -> (-5.6675, 2.1369)
  line L544 (-5.6675, 2.1369) -> (-5.6389, 2.1573)
  line L545 (-5.6389, 2.1573) -> (-5.6137, 2.1798)
  line L546 (-5.6137, 2.1798) -> (-5.5919, 2.2042)
  line L547 (-5.5919, 2.2042) -> (-5.5736, 2.2304)
  line L548 (-5.5736, 2.2304) -> (-5.5559, 2.2655)
  line L549 (-5.5559, 2.2655) -> (-5.4804, 2.4424)
  line L550 (-5.4804, 2.4424) -> (-5.3993, 2.6168)
  line L551 (-5.3993, 2.6168) -> (-5.3851, 2.6535)
  line L552 (-5.3851, 2.6535) -> (-5.3778, 2.6846)
  line L553 (-5.3778, 2.6846) -> (-5.3742, 2.7171)
  line L554 (-5.3742, 2.7171) -> (-5.3743, 2.7508)
  line L555 (-5.3743, 2.7508) -> (-5.3783, 2.7857)
  line L556 (-5.3783, 2.7857) -> (-5.386, 2.8216)
  line L557 (-5.386, 2.8216) -> (-5.3977, 2.8583)
  line L558 (-5.3977, 2.8583) -> (-5.4133, 2.8957)
  line L559 (-5.4133, 2.8957) -> (-5.4328, 2.9336)
  line L560 (-5.4328, 2.9336) -> (-5.4564, 2.9719)
  line L561 (-5.4564, 2.9719) -> (-5.5154, 3.049)
  line L562 (-5.5154, 3.049) -> (-5.5907, 3.1259)
  line L563 (-5.5907, 3.1259) -> (-5.6821, 3.2013)
  line L564 (-5.6821, 3.2013) -> (-5.7897, 3.274)
  line L565 (-5.7897, 3.274) -> (-5.9134, 3.3427)
  line L566 (-5.9134, 3.3427) -> (-6.053, 3.4063)
  line L567 (-6.053, 3.4063) -> (-6.1898, 3.4581)
  line L568 (-6.1898, 3.4581) -> (-6.2836, 3.5337)
  line L569 (-6.2836, 3.5337) -> (-6.3924, 3.6388)
  line L570 (-6.3924, 3.6388) -> (-6.4557, 3.7078)
  line L571 (-6.4557, 3.7078) -> (-6.5237, 3.7885)
  line L572 (-6.5237, 3.7885) -> (-6.5973, 3.8837)
  line L573 (-6.5973, 3.8837) -> (-6.673, 3.9905)
  line L574 (-6.673, 3.9905) -> (-6.7513, 4.1114)
  line L575 (-6.7513, 4.1114) -> (-6.8306, 4.246)
  line L576 (-6.8306, 4.246) -> (-6.9099, 4.3945)
  line L577 (-6.9099, 4.3945) -> (-6.9888, 4.5583)
  line L578 (-6.9888, 4.5583) -> (-7.0627, 4.7295)
  arc A9 (-6.6798, 5.2564) -> (-7.0627, 4.7295) centre (0, 0) ccw
  line L579 (-6.6798, 5.2564) -> (-6.4942, 5.2391)
  line L580 (-6.4942, 5.2391) -> (-6.314, 5.2146)
  line L581 (-6.314, 5.2146) -> (-6.1482, 5.185)
  line L582 (-6.1482, 5.185) -> (-5.9958, 5.1511)
  line L583 (-5.9958, 5.1511) -> (-5.8566, 5.1139)
  line L584 (-5.8566, 5.1139) -> (-5.7316, 5.0749)
  line L585 (-5.7316, 5.0749) -> (-5.6184, 5.0343)
  line L586 (-5.6184, 5.0343) -> (-5.5207, 4.9945)
  line L587 (-5.5207, 4.9945) -> (-5.4355, 4.9557)
  line L588 (-5.4355, 4.9557) -> (-5.3019, 4.8846)
  line L589 (-5.3019, 4.8846) -> (-5.2011, 4.8186)
  line L590 (-5.2011, 4.8186) -> (-5.1095, 4.7045)
  line L591 (-5.1095, 4.7045) -> (-5.006, 4.5914)
  line L592 (-5.006, 4.5914) -> (-4.9024, 4.4949)
  line L593 (-4.9024, 4.4949) -> (-4.8001, 4.415)
  line L594 (-4.8001, 4.415) -> (-4.7001, 4.3513)
  line L595 (-4.7001, 4.3513) -> (-4.6038, 4.3035)
  line L596 (-4.6038, 4.3035) -> (-4.5122, 4.2712)
  line L597 (-4.5122, 4.2712) -> (-4.4685, 4.2606)
  line L598 (-4.4685, 4.2606) -> (-4.4264, 4.2537)
  line L599 (-4.4264, 4.2537) -> (-4.386, 4.2505)
  line L600 (-4.386, 4.2505) -> (-4.3475, 4.2507)
  line L601 (-4.3475, 4.2507) -> (-4.311, 4.2544)
  line L602 (-4.311, 4.2544) -> (-4.2765, 4.2614)
  line L603 (-4.2765, 4.2614) -> (-4.2444, 4.2717)
  line L604 (-4.2444, 4.2717) -> (-4.2146, 4.2851)
  line L605 (-4.2146, 4.2851) -> (-4.1872, 4.3017)
  line L606 (-4.1872, 4.3017) -> (-4.1567, 4.3265)
  line L607 (-4.1567, 4.3265) -> (-4.0159, 4.4575)
  line L608 (-4.0159, 4.4575) -> (-3.8709, 4.5838)
  line L609 (-3.8709, 4.5838) -> (-3.843, 4.6116)
  line L610 (-3.843, 4.6116) -> (-3.8237, 4.637)
  line L611 (-3.8237, 4.637) -> (-3.8072, 4.6653)
  line L612 (-3.8072, 4.6653) -> (-3.7936, 4.6962)
  line L613 (-3.7936, 4.6962) -> (-3.7831, 4.7297)
  line L614 (-3.7831, 4.7297) -> (-3.7756, 4.7656)
  line L615 (-3.7756, 4.7656) -> (-3.7713, 4.8039)
  line L616 (-3.7713, 4.8039) -> (-3.7707, 4.8449)
  line L617 (-3.7707, 4.8449) -> (-3.7731, 4.8875)
  line L618 (-3.7731, 4.8875) -> (-3.7791, 4.9321)
  line L619 (-3.7791, 4.9321) -> (-3.8017, 5.0266)
  line L620 (-3.8017, 5.0266) -> (-3.8392, 5.1274)
  line L621 (-3.8392, 5.1274) -> (-3.892, 5.2334)
  line L622 (-3.892, 5.2334) -> (-3.9608, 5.3436)
  line L623 (-3.9608, 5.3436) -> (-4.0459, 5.4566)
  line L624 (-4.0459, 5.4566) -> (-4.1476, 5.5714)
  line L625 (-4.1476, 5.5714) -> (-4.2515, 5.6744)
  line L626 (-4.2515, 5.6744) -> (-4.3066, 5.7816)
  line L627 (-4.3066, 5.7816) -> (-4.3633, 5.9219)
  line L628 (-4.3633, 5.9219) -> (-4.393, 6.0106)
  line L629 (-4.393, 6.0106) -> (-4.4224, 6.112)
  line L630 (-4.4224, 6.112) -> (-4.451, 6.2289)
  line L631 (-4.451, 6.2289) -> (-4.4767, 6.3572)
  line L632 (-4.4767, 6.3572) -> (-4.4991, 6.4995)
  line L633 (-4.4991, 6.4995) -> (-4.5168, 6.6547)
  line L634 (-4.5168, 6.6547) -> (-4.529, 6.8226)
  line L635 (-4.529, 6.8226) -> (-4.5345, 7.0044)
  line L636 (-4.5345, 7.0044) -> (-4.5323, 7.1908)
  arc A10 (-3.963, 7.5196) -> (-4.5323, 7.1908) centre (0, 0) ccw
  line L637 (-3.963, 7.5196) -> (-3.8005, 7.4283)
  line L638 (-3.8005, 7.4283) -> (-3.6458, 7.3326)
  line L639 (-3.6458, 7.3326) -> (-3.5065, 7.2381)
  line L640 (-3.5065, 7.2381) -> (-3.381, 7.1451)
  line L641 (-3.381, 7.1451) -> (-3.2689, 7.0546)
  line L642 (-3.2689, 7.0546) -> (-3.1706, 6.9681)
  line L643 (-3.1706, 6.9681) -> (-3.0837, 6.885)
  line L644 (-3.0837, 6.885) -> (-3.0106, 6.8089)
  line L645 (-3.0106, 6.8089) -> (-2.9485, 6.7387)
  line L646 (-2.9485, 6.7387) -> (-2.8554, 6.6195)
  line L647 (-2.8554, 6.6195) -> (-2.7901, 6.5182)
  line L648 (-2.7901, 6.5182) -> (-2.7529, 6.3768)
  line L649 (-2.7529, 6.3768) -> (-2.7043, 6.2313)
  line L650 (-2.7043, 6.2313) -> (-2.6489, 6.1011)
  line L651 (-2.6489, 6.1011) -> (-2.5879, 5.9864)
  line L652 (-2.5879, 5.9864) -> (-2.5225, 5.8876)
  line L653 (-2.5225, 5.8876) -> (-2.4539, 5.8048)
  line L654 (-2.4539, 5.8048) -> (-2.3834, 5.7379)
  line L655 (-2.3834, 5.7379) -> (-2.3478, 5.7105)
  line L656 (-2.3478, 5.7105) -> (-2.3121, 5.6871)
  line L657 (-2.3121, 5.6871) -> (-2.2765, 5.6677)
  line L658 (-2.2765, 5.6677) -> (-2.2413, 5.6522)
  line L659 (-2.2413, 5.6522) -> (-2.2064, 5.6407)
  line L660 (-2.2064, 5.6407) -> (-2.1721, 5.6332)
  line L661 (-2.1721, 5.6332) -> (-2.1385, 5.6295)
  line L662 (-2.1385, 5.6295) -> (-2.1058, 5.6297)
  line L663 (-2.1058, 5.6297) -> (-2.0742, 5.6336)
  line L664 (-2.0742, 5.6336) -> (-2.0362, 5.6439)
  line L665 (-2.0362, 5.6439) -> (-1.8543, 5.7063)
  line L666 (-1.8543, 5.7063) -> (-1.6704, 5.7628)
  line L667 (-1.6704, 5.7628) -> (-1.6337, 5.7768)
  line L668 (-1.6337, 5.7768) -> (-1.6057, 5.7922)
  line L669 (-1.6057, 5.7922) -> (-1.5791, 5.8113)
  line L670 (-1.5791, 5.8113) -> (-1.5541, 5.834)
  line L671 (-1.5541, 5.834) -> (-1.5308, 5.8603)
  line L672 (-1.5308, 5.8603) -> (-1.5094, 5.8901)
  line L673 (-1.5094, 5.8901) -> (-1.4899, 5.9233)
  line L674 (-1.4899, 5.9233) -> (-1.4726, 5.96)
  line L675 (-1.4726, 5.96) -> (-1.4575, 5.9999)
  line L676 (-1.4575, 5.9999) -> (-1.4448, 6.043)
  line L677 (-1.4448, 6.043) -> (-1.427, 6.1385)
  line L678 (-1.427, 6.1385) -> (-1.4203, 6.2459)
  line L679 (-1.4203, 6.2459) -> (-1.4255, 6.3642)
  line L680 (-1.4255, 6.3642) -> (-1.4435, 6.4928)
  line L681 (-1.4435, 6.4928) -> (-1.4752, 6.6307)
  line L682 (-1.4752, 6.6307) -> (-1.5215, 6.777)
  line L683 (-1.5215, 6.777) -> (-1.5745, 6.9133)
  line L684 (-1.5745, 6.9133) -> (-1.5813, 7.0336)
  line L685 (-1.5813, 7.0336) -> (-1.576, 7.1848)
  line L686 (-1.576, 7.1848) -> (-1.5671, 7.278)
  line L687 (-1.5671, 7.278) -> (-1.5527, 7.3826)
  line L688 (-1.5527, 7.3826) -> (-1.5312, 7.5009)
  line L689 (-1.5312, 7.5009) -> (-1.5025, 7.6286)
  line L690 (-1.5025, 7.6286) -> (-1.4651, 7.7678)
  line L691 (-1.4651, 7.7678) -> (-1.4182, 7.9167)
  line L692 (-1.4182, 7.9167) -> (-1.361, 8.0751)
  line L693 (-1.361, 8.0751) -> (-1.2921, 8.2434)
  line L694 (-1.2921, 8.2434) -> (-1.2143, 8.4128)
  arc A11 (-0.562, 8.4814) -> (-1.2143, 8.4128) centre (0, 0) ccw
  line L695 (-0.562, 8.4814) -> (-0.4507, 8.3318)
  line L696 (-0.4507, 8.3318) -> (-0.3483, 8.1815)
  line L697 (-0.3483, 8.1815) -> (-0.2595, 8.0385)
  line L698 (-0.2595, 8.0385) -> (-0.1826, 7.9026)
  line L699 (-0.1826, 7.9026) -> (-0.1171, 7.7742)
  line L700 (-0.1171, 7.7742) -> (-0.0625, 7.6553)
  line L701 (-0.0625, 7.6553) -> (-0.0169, 7.544)
  line L702 (-0.0169, 7.544) -> (0.0189, 7.4447)
  line L703 (0.0189, 7.4447) -> (0.0471, 7.3554)
  line L704 (0.0471, 7.3554) -> (0.0837, 7.2086)
  line L705 (0.0837, 7.2086) -> (0.1021, 7.0895)
  line L706 (0.1021, 7.0895) -> (0.0786, 6.9451)
  line L707 (0.0786, 6.9451) -> (0.0637, 6.7924)
  line L708 (0.0637, 6.7924) -> (0.0614, 6.651)
  line L709 (0.0614, 6.651) -> (0.0705, 6.5214)
  line L710 (0.0705, 6.5214) -> (0.09, 6.4046)
  line L711 (0.09, 6.4046) -> (0.119, 6.301)
  line L712 (0.119, 6.301) -> (0.1562, 6.2112)
  line L713 (0.1562, 6.2112) -> (0.1776, 6.1717)
  line L714 (0.1776, 6.1717) -> (0.2007, 6.1358)
  line L715 (0.2007, 6.1358) -> (0.2253, 6.1036)
  line L716 (0.2253, 6.1036) -> (0.2512, 6.0751)
  line L717 (0.2512, 6.0751) -> (0.2784, 6.0505)
  line L718 (0.2784, 6.0505) -> (0.3066, 6.0296)
  line L719 (0.3066, 6.0296) -> (0.3358, 6.0126)
  line L720 (0.3358, 6.0126) -> (0.3657, 5.9994)
  line L721 (0.3657, 5.9994) -> (0.3963, 5.9902)
  line L722 (0.3963, 5.9902) -> (0.4352, 5.9841)
  line L723 (0.4352, 5.9841) -> (0.6267, 5.9671)
  line L724 (0.6267, 5.9671) -> (0.8176, 5.9439)
  line L725 (0.8176, 5.9439) -> (0.8569, 5.9417)
  line L726 (0.8569, 5.9417) -> (0.8888, 5.9444)
  line L727 (0.8888, 5.9444) -> (0.9208, 5.9511)
  line L728 (0.9208, 5.9511) -> (0.9529, 5.9617)
  line L729 (0.9529, 5.9617) -> (0.9848, 5.9762)
  line L730 (0.9848, 5.9762) -> (1.0165, 5.9947)
  line L731 (1.0165, 5.9947) -> (1.0478, 6.0172)
  line L732 (1.0478, 6.0172) -> (1.0786, 6.0436)
  line L733 (1.0786, 6.0436) -> (1.1086, 6.0739)
  line L734 (1.1086, 6.0739) -> (1.1377, 6.1081)
  line L735 (1.1377, 6.1081) -> (1.1928, 6.1881)
  line L736 (1.1928, 6.1881) -> (1.2427, 6.2834)
  line L737 (1.2427, 6.2834) -> (1.2861, 6.3937)
  line L738 (1.2861, 6.3937) -> (1.3219, 6.5185)
  line L739 (1.3219, 6.5185) -> (1.349, 6.6574)
  line L740 (1.349, 6.6574) -> (1.3663, 6.8098)
  line L741 (1.3663, 6.8098) -> (1.3733, 6.9559)
  line L742 (1.3733, 6.9559) -> (1.416, 7.0686)
  line L743 (1.416, 7.0686) -> (1.4823, 7.2045)
  line L744 (1.4823, 7.2045) -> (1.5284, 7.286)
  line L745 (1.5284, 7.286) -> (1.5841, 7.3757)
  line L746 (1.5841, 7.3757) -> (1.6519, 7.4751)
  line L747 (1.6519, 7.4751) -> (1.73, 7.5801)
  line L748 (1.73, 7.5801) -> (1.8208, 7.692)
  line L749 (1.8208, 7.692) -> (1.9242, 7.809)
  line L750 (1.9242, 7.809) -> (2.0409, 7.9304)
  line L751 (2.0409, 7.9304) -> (2.1724, 8.0563)
  line L752 (2.1724, 8.0563) -> (2.3123, 8.1794)
  arc A12 (2.9364, 7.9767) -> (2.3123, 8.1794) centre (0, 0) ccw
  line L753 (2.9364, 7.9767) -> (2.9773, 7.7948)
  line L754 (2.9773, 7.7948) -> (3.0097, 7.6158)
  line L755 (3.0097, 7.6158) -> (3.0327, 7.449)
  line L756 (3.0327, 7.449) -> (3.0476, 7.2936)
  line L757 (3.0476, 7.2936) -> (3.0553, 7.1497)
  line L758 (3.0553, 7.1497) -> (3.0568, 7.0188)
  line L759 (3.0568, 7.0188) -> (3.0531, 6.8986)
  line L760 (3.0531, 6.8986) -> (3.0455, 6.7933)
  line L761 (3.0455, 6.7933) -> (3.0349, 6.7003)
  line L762 (3.0349, 6.7003) -> (3.0086, 6.5513)
  line L763 (3.0086, 6.5513) -> (2.977, 6.435)
  line L764 (2.977, 6.435) -> (2.8968, 6.3127)
  line L765 (2.8968, 6.3127) -> (2.8212, 6.1792)
  line L766 (2.8212, 6.1792) -> (2.7615, 6.0509)
  line L767 (2.7615, 6.0509) -> (2.7171, 5.9289)
  line L768 (2.7171, 5.9289) -> (2.6874, 5.8142)
  line L769 (2.6874, 5.8142) -> (2.6717, 5.7078)
  line L770 (2.6717, 5.7078) -> (2.6693, 5.6106)
  line L771 (2.6693, 5.6106) -> (2.6727, 5.5658)
  line L772 (2.6727, 5.5658) -> (2.6792, 5.5237)
  line L773 (2.6792, 5.5237) -> (2.6885, 5.4843)
  line L774 (2.6885, 5.4843) -> (2.7007, 5.4477)
  line L775 (2.7007, 5.4477) -> (2.7154, 5.4141)
  line L776 (2.7154, 5.4141) -> (2.7328, 5.3835)
  line L777 (2.7328, 5.3835) -> (2.7525, 5.3561)
  line L778 (2.7525, 5.3561) -> (2.7745, 5.3319)
  line L779 (2.7745, 5.3319) -> (2.7987, 5.311)
  line L780 (2.7987, 5.311) -> (2.8317, 5.2897)
  line L781 (2.8317, 5.2897) -> (2.9998, 5.1962)
  line L782 (2.9998, 5.1962) -> (3.1648, 5.0974)
  line L783 (3.1648, 5.0974) -> (3.1998, 5.0795)
  line L784 (3.1998, 5.0795) -> (3.23, 5.069)
  line L785 (3.23, 5.069) -> (3.2619, 5.062)
  line L786 (3.2619, 5.062) -> (3.2955, 5.0586)
  line L787 (3.2955, 5.0586) -> (3.3306, 5.0589)
  line L788 (3.3306, 5.0589) -> (3.3671, 5.0629)
  line L789 (3.3671, 5.0629) -> (3.4048, 5.0707)
  line L790 (3.4048, 5.0707) -> (3.4437, 5.0823)
  line L791 (3.4437, 5.0823) -> (3.4834, 5.0978)
  line L792 (3.4834, 5.0978) -> (3.524, 5.1172)
  line L793 (3.524, 5.1172) -> (3.6068, 5.1679)
  line L794 (3.6068, 5.1679) -> (3.6911, 5.2347)
  line L795 (3.6911, 5.2347) -> (3.7757, 5.3178)
  line L796 (3.7757, 5.3178) -> (3.8591, 5.4172)
  line L797 (3.8591, 5.4172) -> (3.9404, 5.5331)
  line L798 (3.9404, 5.5331) -> (4.0181, 5.6653)
  line L799 (4.0181, 5.6653) -> (4.084, 5.796)
  line L800 (4.084, 5.796) -> (4.1688, 5.8815)
  line L801 (4.1688, 5.8815) -> (4.2847, 5.9787)
  line L802 (4.2847, 5.9787) -> (4.36, 6.0344)
  line L803 (4.36, 6.0344) -> (4.4473, 6.0937)
  line L804 (4.4473, 6.0937) -> (4.5496, 6.157)
  line L805 (4.5496, 6.157) -> (4.6637, 6.2211)
  line L806 (4.6637, 6.2211) -> (4.7922, 6.2864)
  line L807 (4.7922, 6.2864) -> (4.9343, 6.3512)
  line L808 (4.9343, 6.3512) -> (5.0902, 6.4147)
  line L809 (5.0902, 6.4147) -> (5.2614, 6.4761)
  line L810 (5.2614, 6.4761) -> (5.4394, 6.5316)
  arc A13 (5.9268, 6.0928) -> (5.4394, 6.5316) centre (0, 0) ccw
  line L811 (5.9268, 6.0928) -> (5.8902, 5.91)
  line L812 (5.8902, 5.91) -> (5.847, 5.7334)
  line L813 (5.847, 5.7334) -> (5.8002, 5.5716)
  line L814 (5.8002, 5.5716) -> (5.7506, 5.4236)
  line L815 (5.7506, 5.4236) -> (5.699, 5.289)
  line L816 (5.699, 5.289) -> (5.6472, 5.1688)
  line L817 (5.6472, 5.1688) -> (5.595, 5.0605)
  line L818 (5.595, 5.0605) -> (5.5452, 4.9674)
  line L819 (5.5452, 4.9674) -> (5.4977, 4.8867)
  line L820 (5.4977, 4.8867) -> (5.4131, 4.7613)
  line L821 (5.4131, 4.7613) -> (5.3369, 4.6679)
  line L822 (5.3369, 4.6679) -> (5.2139, 4.5888)
  line L823 (5.2139, 4.5888) -> (5.0905, 4.4976)
  line L824 (5.0905, 4.4976) -> (4.9838, 4.4047)
  line L825 (4.9838, 4.4047) -> (4.8936, 4.3113)
  line L826 (4.8936, 4.3113) -> (4.8198, 4.2186)
  line L827 (4.8198, 4.2186) -> (4.7622, 4.1277)
  line L828 (4.7622, 4.1277) -> (4.7204, 4.04)
  line L829 (4.7204, 4.04) -> (4.7054, 3.9976)
  line L830 (4.7054, 3.9976) -> (4.6941, 3.9565)
  line L831 (4.6941, 3.9565) -> (4.6867, 3.9167)
  line L832 (4.6867, 3.9167) -> (4.6829, 3.8784)
  line L833 (4.6829, 3.8784) -> (4.6827, 3.8417)
  line L834 (4.6827, 3.8417) -> (4.6861, 3.8067)
  line L835 (4.6861, 3.8067) -> (4.6929, 3.7736)
  line L836 (4.6929, 3.7736) -> (4.7032, 3.7426)
  line L837 (4.7032, 3.7426) -> (4.7168, 3.7137)
  line L838 (4.7168, 3.7137) -> (4.7383, 3.6807)
  line L839 (4.7383, 3.6807) -> (4.8538, 3.527)
  line L840 (4.8538, 3.527) -> (4.9644, 3.3696)
  line L841 (4.9644, 3.3696) -> (4.9891, 3.339)
  line L842 (4.9891, 3.339) -> (5.0124, 3.3171)
  line L843 (5.0124, 3.3171) -> (5.0387, 3.2977)
  line L844 (5.0387, 3.2977) -> (5.068, 3.281)
  line L845 (5.068, 3.281) -> (5.1002, 3.267)
  line L846 (5.1002, 3.267) -> (5.1352, 3.2558)
  line L847 (5.1352, 3.2558) -> (5.1728, 3.2476)
  line L848 (5.1728, 3.2476) -> (5.213, 3.2424)
  line L849 (5.213, 3.2424) -> (5.2556, 3.2404)
  line L850 (5.2556, 3.2404) -> (5.3006, 3.2416)
  line L851 (5.3006, 3.2416) -> (5.3969, 3.2542)
  line L852 (5.3969, 3.2542) -> (5.5011, 3.2809)
  line L853 (5.5011, 3.2809) -> (5.6121, 3.3225)
  line L854 (5.6121, 3.3225) -> (5.7288, 3.3793)
  line L855 (5.7288, 3.3793) -> (5.8501, 3.4521)
  line L856 (5.8501, 3.4521) -> (5.9749, 3.5413)
  line L857 (5.9749, 3.5413) -> (6.0882, 3.6339)
  line L858 (6.0882, 3.6339) -> (6.2005, 3.6775)
  line L859 (6.2005, 3.6775) -> (6.346, 3.7192)
  line L860 (6.346, 3.7192) -> (6.4374, 3.7395)
  line L861 (6.4374, 3.7395) -> (6.5413, 3.7581)
  line L862 (6.5413, 3.7581) -> (6.6605, 3.7743)
  line L863 (6.6605, 3.7743) -> (6.7908, 3.7864)
  line L864 (6.7908, 3.7864) -> (6.9347, 3.7938)
  line L865 (6.9347, 3.7938) -> (7.0909, 3.7953)
  line L866 (7.0909, 3.7953) -> (7.2591, 3.7898)
  line L867 (7.2591, 3.7898) -> (7.4406, 3.7763)
  line L868 (7.4406, 3.7763) -> (7.6258, 3.7547)
  arc A14 (7.8927, 3.1553) -> (7.6258, 3.7547) centre (0, 0) ccw
  line L869 (7.8927, 3.1553) -> (7.7848, 3.0032)
  line L870 (0, 3.4641) -> (3, 1.7321)
  line L871 (3, 1.7321) -> (3, -1.7321)
  line L872 (3, -1.7321) -> (0, -3.4641)
  line L873 (0, -3.4641) -> (-3, -1.7321)
  line L874 (-3, -1.7321) -> (-3, 1.7321)
  line L875 (-3, 1.7321) -> (0, 3.4641)
  point P0 (3, 0)
  dimension "d0" = 6
  constraints: 1752 end point, 30 parallel, 30 point on circle, 20 concentric, 15 centre point, 2 coincident, 1 horizontal alignment, 1 midpoint, 13 other
  measures "d0" distance of L871.end L873.end
extrude "Extrusión1" add sketch "Boceto1" along normal blind 6
